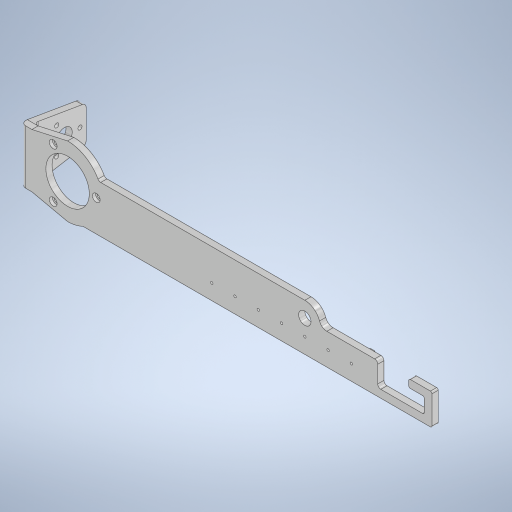
# Autodesk Inventor part: motor_holder_2
Saved by Autodesk Inventor 2024 (Build 280153000, 153)
## iProperties
Created: 2025-02-07
Part Number: motor_holder_2
Material: アルミニウム 6061
Document SubType Name: Modeling
Designer: 1412z
Density: 2.7 g/cm^3
Appearance: アルミニウム - つや出し
Author: 1412z
Autodesk Inventor part; units mm, degrees
ref_plane "YZ Plane" through (0, 0, 0) normal (1, 0, 0) x (0, 1, 0)
ref_plane "XZ Plane" through (0, 0, 0) normal (0, 1, 0) x (-1, 0, 0)
ref_plane "XY Plane" through (0, 0, 0) normal (0, 0, 1) x (1, 0, 0)
sketch "スケッチ1" plane through (0, 0, 0) normal (1, 0, 0) x (0, 1, 0)
  circle A0 centre (0, 0) radius 10
  circle A1 centre (0, -10) radius 1.35
  circle A2 centre (8.6603, 5) radius 1.35
  circle A3 centre (-8.6603, 5) radius 1.35
  circle A4 centre (0, 0) radius 5
  line L0 (0, 0) -> (0, 50)
  circle A5 centre (0, 50) radius 22.5
  circle A6 centre (0, 0) radius 14
  line L1 (-14, 0) -> (-22.5, 50)
  line L2 (14, 0) -> (22.5, 50)
  line L3 (0, -14) -> (-11.62, -14)
  line L4 (-11.62, -14) -> (-14, 0)
  line L5 (0, -14) -> (11.62, -14)
  line L6 (11.62, -14) -> (14, 0)
  line L7 (0, 20) -> (-17.4, 20)
  line L8 (0, 20) -> (17.4, 20)
  dimension "d0" = 20
  dimension "d1" = 2.7
  dimension "d4" = 360
  dimension "d6" = 10
  dimension "d7" = 50
  dimension "d8" = 45
  dimension "d9" = 28
  constraints: 18 end point, 7 point on line, 6 centre point, 6 coincident, 5 point on circle, 1 horizontal, 1 perpendicular, 1 tangent, 1 vertical, 1 vertical alignment, 10 other
  measures "d1" diameter of A1
  measures "d6" diameter of A4
  measures "d7" distance of L0.start L0.end
  measures "d8" diameter of A5
  measures "d9" diameter of A6
extrude "押し出し1" add sketch "スケッチ1" along normal blind 4 contours A0 A1 A3 A2 | A6 L1 L7 L0 | L0 L8 L2 A6 | A6 L6 L4 | L6 L5 A6 | A6 L3 L4
sketch "スケッチ2" plane through (0, -17.4, 20) normal (0, 0, 1) x (1, 0, 0)
  line L0 (0, 17.4) -> (30, 17.4)
  circle A0 centre (30, 17.4) radius 22.5
  circle A1 centre (30, 17.4) radius 18.5
  circle A2 centre (30, 17.4) radius 14
  circle A3 centre (48.5, 17.4) radius 1.35
  circle A4 centre (20.75, 33.4215) radius 1.35
  circle A5 centre (20.75, 1.3785) radius 1.35
  line L1 (0, 29.02) -> (0, 34.8) projected
  line L2 (0, 0) -> (0, 5.78) projected
  line L3 (0, 34.8) -> (0, 0)
  line L4 (4, 29.02) -> (4, 34.8) projected
  line L5 (4, 34.8) -> (7, 34.8)
  line L6 (7, 34.8) -> (30, 39.9)
  line L7 (4, 0) -> (4, 5.78) projected
  line L8 (4, 0) -> (7, 0)
  line L9 (7, 0) -> (30, -5.1)
  line L10 (4, 0) -> (0, 0)
  line L11 (0, 34.8) -> (4, 34.8) projected
  line L12 (0, 0) -> (0, 34.8)
  line L13 (0, 34.8) -> (4, 34.8)
  dimension "d14" = 37
  dimension "d12" = 30
  dimension "d13" = 45
  dimension "d15" = 28
  dimension "d16" = 2.7
  dimension "d19" = 360
  dimension "d21" = 3
  dimension "d22" = 3
  constraints: 18 end point, 5 centre point, 4 horizontal, 3 coincident, 2 point on circle, 1 collinear, 1 horizontal alignment, 1 perpendicular, 1 vertical, 9 other
  measures "d12" distance of L0.start L0.end
  measures "d13" diameter of A0
  measures "d15" diameter of A2
  measures "d16" diameter of A3
  measures "d21" distance of L4.end L5.end
  measures "d22" distance of L7.start L8.end
extrude "押し出し2" add sketch "スケッチ2" along normal blind 4 contours L3 L1 L11 L5 L6 A0 L0 | L0 A0 L9 L8 L10 L2 L3 | A0 L6 L9 | A3 A1 A5 A4
fillet "フィレット1" radius 3 2 edges at (4, 0, 20) (0, 0, 24)
fillet "フィレット2" radius 3 2 edges at (2, -11.62, -14) (2, 11.62, -14)
sketch "スケッチ7" plane through (0, -17.4, 24) normal (0, 0, 1) x (1, 0, 0)
  circle A0 centre (30, 17.4) radius 14 projected
  line L0 (30, 17.4) -> (182.95, 17.4)
  line L1 (30, 17.4) -> (182.95, 17.4) construction
  circle A1 centre (182.95, 17.4) radius 4
  circle A2 centre (182.95, 17.4) radius 10
  line L2 (182.95, 27.4) -> (50.1556, 27.4)
  arc A3 (30, -5.1) -> (30, 39.9) centre (30, 17.4) ccw projected
  line L3 (182.95, 27.4) -> (315.7444, 27.4) construction
  line L4 (182.95, 7.4) -> (50.1556, 7.4)
  point P0 (0, 17.4)
  dimension "d55" = 152.95
  dimension "d56" = 0
  dimension "d57" = 8
  dimension "d58" = 20
  dimension "d59" = 180
  constraints: 10 end point, 4 horizontal, 4 point on circle, 2 centre point, 2 coincident, 2 collinear, 1 tangent
  measures "d55" distance of L0.start L0.end
  measures "d56" distance between parallel lines of L0 L1
  measures "d57" diameter of A1
  measures "d58" diameter of A2
  measures "d59" angle of L2 L3
extrude "押し出し7" add sketch "スケッチ7" against normal blind 4 contours A3 L2 A2 L0 | L0 A2 L4 A3 | A2
fillet "フィレット3" radius 2 2 edges at (50.1556, 10, 22) (50.1556, -10, 22)
sketch "スケッチ8" plane through (0, -17.4, 24) normal (0, 0, 1) x (1, 0, 0)
  circle A0 centre (20.75, 33.4215) radius 1.35 projected
  circle A1 centre (20.75, 33.4215) radius 2.5
  circle A2 centre (48.5, 17.4) radius 1.35 projected
  circle A3 centre (48.5, 17.4) radius 2.5
  circle A4 centre (20.75, 1.3785) radius 1.35 projected
  circle A5 centre (20.75, 1.3785) radius 2.5
  point P0 (0, 17.4)
  dimension "d63" = 5
  dimension "d64" = 5
  dimension "d65" = 5
  constraints: 3 centre point, 3 coincident
  measures "d63" diameter of A1
  measures "d64" diameter of A3
  measures "d65" diameter of A5
extrude "押し出し8" cut sketch "スケッチ8" against normal blind 2 contours A0 | A1 | A3 | A4 | A5
sketch "スケッチ9" plane through (0, -17.4, 24) normal (0, 0, 1) x (1, 0, 0)
  circle A0 centre (182.95, 17.4) radius 4 projected
  line L0 (182.95, 17.4) -> (182.95, -2.8)
  line L1 (182.95, -2.8) -> (229.95, -2.8)
  line L2 (229.95, -2.8) -> (229.95, 17.2)
  arc A1 (182.95, 7.4) -> (182.95, 27.4) centre (182.95, 17.4) ccw projected
  line L3 (229.95, -2.8) -> (264.95, -2.8)
  line L4 (264.95, -2.8) -> (264.95, 17.2)
  line L5 (264.95, 17.2) -> (249.95, 17.2)
  line L6 (249.95, 17.2) -> (249.95, 12.2)
  line L7 (182.95, -2.8) -> (39.9101, -2.8)
  arc A2 (30, -5.1) -> (49.6163, 6.3796) centre (30, 17.4) ccw projected
  circle A3 centre (30, 17.4) radius 14 projected
  circle A4 centre (30, 17.4) radius 22.5
  arc A5 (49.6163, 28.4204) -> (51.36, 27.4) centre (51.36, 29.4) ccw projected
  circle A6 centre (51.36, 29.4) radius 2
  line L8 (51.36, 27.4) -> (182.95, 27.4) projected
  line L9 (51.36, 27.4) -> (182.95, 27.4)
  circle A7 centre (182.95, 17.4) radius 10
  line L10 (229.95, 17.2) -> (192.948, 17.2)
  line L11 (249.95, 12.2) -> (259.95, 12.2)
  line L12 (259.95, 12.2) -> (259.95, 2.2)
  line L13 (259.95, 2.2) -> (229.95, 2.2)
  point P0 (0, 17.4)
  point P1 (182.95, 7.4)
  point P2 (182.95, 27.4)
  point P3 (49.6163, 6.3796)
  dimension "d68" = 20.2
  dimension "d69" = 47
  dimension "d70" = 20
  dimension "d71" = 35
  dimension "d72" = 20
  dimension "d73" = 15
  dimension "d74" = 5
  dimension "d76" = 10
  dimension "d77" = 10
  constraints: 26 end point, 5 horizontal, 5 perpendicular, 3 coincident, 2 vertical, 1 centre point, 1 collinear, 1 point on circle, 1 point on line, 1 tangent, 7 other
  measures "d68" distance of L0.start L0.end
  measures "d69" distance of L0.end L1.end
  measures "d70" distance of L1.end L2.end
  measures "d71" distance of L1.end L3.end
  measures "d72" distance of L3.end L4.end
  measures "d73" distance of L4.end L5.end
  measures "d74" distance of L5.end L6.end
  measures "d76" distance of L6.end L11.end
  measures "d77" distance of L11.end L12.end
extrude "押し出し9" add sketch "スケッチ9" against normal blind 4 contours A1 L10 L2 L1 L0 | L0 L7 A2 A4 A5 L8 A7 | L2 L13 L12 L11 L6 L5 L4 L3
fillet "フィレット7" radius 5 1 edges at (192.948, -0.2, 22)
fillet "フィレット8" radius 2 2 edges at (39.9101, -20.2, 22) (229.95, -0.2, 22)
fillet "フィレット9" radius 2 1 edges at (229.95, -15.2, 22)
fillet "フィレット10" radius 1 6 edges at (249.95, -0.2, 22) (249.95, -5.2, 22) (259.95, -5.2, 22) (259.95, -15.2, 22) (264.95, -0.2, 22) (264.95, -20.2, 22)
sketch "スケッチ14" plane through (0, -17.4, 20) normal (0, 0, -1) x (-1, 0, 0)
  line L0 (-229.95, 15.2) -> (-229.95, 4.2) projected
  line L1 (-229.95, 7.1) -> (-229.95, 9.7)
  line L2 (-229.95, 9.7) -> (-117.95, 9.7)
  line L3 (-117.95, 9.7) -> (-117.95, 4.5)
  line L4 (-117.95, 4.5) -> (-229.95, 4.5)
  line L5 (-229.95, 4.5) -> (-229.95, 7.1)
  point P0 (0, 17.4)
  dimension "d116" = 2.6
  dimension "d117" = 112
  dimension "d118" = 5.2
  constraints: 10 end point, 2 perpendicular, 2 point on line, 1 collinear, 1 midpoint, 1 vertical
  measures "d116" distance of L1.start L1.end
  measures "d117" distance of L1.end L2.end
  measures "d118" distance of L2.end L3.end
extrude "押し出し14" cut sketch "スケッチ14" against normal blind 0.7
sketch "スケッチ18" plane through (0, -17.4, 20.7) normal (0, 0, -1) x (-1, 0, 0)
  circle A0 centre (-212.95, 7.1) radius 0.8
  circle A1 centre (-197.95, 7.1) radius 0.8
  circle A2 centre (-182.95, 7.1) radius 0.8
  circle A3 centre (-167.95, 7.1) radius 0.8
  circle A4 centre (-152.95, 7.1) radius 0.8
  circle A5 centre (-137.95, 7.1) radius 0.8
  circle A6 centre (-122.95, 7.1) radius 0.8
  point P0 (0, 17.4)
  dimension "d154" = 1.6
  dimension "d155" = 1.6
  dimension "d156" = 15
  dimension "d157" = 1.6
  dimension "d158" = 15
  dimension "d159" = 1.6
  dimension "d160" = 15
  dimension "d161" = 1.6
  dimension "d162" = 15
  dimension "d163" = 1.6
  dimension "d164" = 15
  dimension "d165" = 1.6
  dimension "d166" = 15
  constraints: 7 centre point
  measures "d154" diameter of A0
  measures "d155" diameter of A1
  measures "d156" distance between centres of A1 A0
  measures "d157" diameter of A2
  measures "d158" distance of A2.centre A1.centre
  measures "d159" diameter of A3
  measures "d160" distance of A3.centre A2.centre
  measures "d161" diameter of A4
  measures "d162" distance of A4.centre A3.centre
  measures "d163" diameter of A5
  measures "d164" distance of A5.centre A4.centre
  measures "d165" diameter of A6
  measures "d166" distance of A6.centre A5.centre
extrude "押し出し18" cut sketch "スケッチ18" against normal blind 10
sketch "スケッチ19" plane through (0, -17.4, 20.7) normal (0, 0, -1) x (-1, 0, 0)
  line L0 (-229.95, 4.5) -> (-229.95, 9.7) projected
  line L1 (-229.95, 4.5) -> (-225.15, 4.5)
  line L2 (-117.95, 4.5) -> (-229.95, 4.5) projected
  line L3 (-225.15, 4.5) -> (-225.15, 9.7)
  line L4 (-229.95, 9.7) -> (-117.95, 9.7) projected
  line L5 (-225.15, 9.7) -> (-229.95, 9.7)
  line L6 (-229.95, 9.7) -> (-229.95, 4.5)
  point P0 (0, 17.4)
  dimension "d169" = 4.8
  constraints: 8 end point, 2 perpendicular, 2 point on line, 1 horizontal
  measures "d169" distance of L0.start L1.end
extrude "押し出し19" add sketch "スケッチ19" along normal blind 0.7
sketch "スケッチ20" plane through (117.95, -12.9, 20) normal (1, 0, 0) x (0, 0, -1)
  line L0 (0, 5.2) -> (0, 0) projected
  line L1 (-0.7, 5.2) -> (-0.7, 0) projected
  line L2 (0, 0) -> (-0.7, 0)
  line L3 (-0.7, 0) -> (-0.7, 5.2)
  line L4 (0, 5.2) -> (-0.7, 5.2) projected
  line L5 (-0.7, 5.2) -> (0, 5.2)
  line L6 (0, 5.2) -> (0, 0)
  point P0 (20, 12.9)
  constraints: 8 end point, 2 collinear, 2 perpendicular
extrude "押し出し20" cut sketch "スケッチ20" against normal blind 0.2
sketch "スケッチ21" plane through (0, -17.4, 20) normal (0, 0, -1) x (-1, 0, 0)
  line L0 (-117.75, 4.5) -> (-225.15, 4.5) projected
  line L1 (-117.75, 4.5) -> (-117.75, -0.5)
  line L2 (-117.75, -0.5) -> (-114.75, -0.5)
  line L3 (-114.75, -0.5) -> (-114.75, 14.5)
  line L4 (-114.75, 14.5) -> (-117.75, 14.5)
  line L5 (-117.75, 14.5) -> (-117.75, 4.5)
  point P0 (0, 17.4)
  dimension "d174" = 5
  dimension "d175" = 3
  dimension "d176" = 15
  constraints: 10 end point, 3 perpendicular, 1 horizontal, 1 vertical
  measures "d174" distance of L0.start L1.end
  measures "d175" distance of L1.end L2.end
  measures "d176" distance of L2.end L3.end
extrude "押し出し21" add sketch "スケッチ21" along normal blind 3
fillet "フィレット13" radius 2 3 edges at (116.25, -17.9, 20) (114.75, -10.4, 20) (116.25, -2.9, 20)
sketch "スケッチ23" plane through (0, -17.4, 20.7) normal (0, 0, -1) x (-1, 0, 0)
  line L0 (-225.15, 9.7) -> (-225.15, 4.5) projected
  line L1 (-225.15, 9.7) -> (-218.15, 9.7)
  line L2 (-225.15, 9.7) -> (-117.75, 9.7) projected
  line L3 (-218.15, 9.7) -> (-218.15, 4.5)
  line L4 (-117.75, 4.5) -> (-225.15, 4.5) projected
  line L5 (-218.15, 4.5) -> (-225.15, 4.5)
  line L6 (-225.15, 4.5) -> (-225.15, 9.7)
  point P0 (0, 17.4)
  dimension "d185" = 7
  constraints: 8 end point, 2 perpendicular, 2 point on line, 1 collinear
  measures "d185" distance of L0.start L1.end
extrude "押し出し23" add sketch "スケッチ23" along normal blind 0.7
sketch "スケッチ26" plane through (0, -17.4, 20) normal (0, 0, -1) x (-1, 0, 0)
  line L0 (-218.15, 9.7) -> (-117.75, 9.7) projected
  line L1 (-218.15, 9.7) -> (-218.15, 14.7)
  line L2 (-218.15, 14.7) -> (-221.15, 14.7)
  line L3 (-221.15, 14.7) -> (-221.15, -0.3)
  line L4 (-221.15, -0.3) -> (-218.15, -0.3)
  line L5 (-218.15, -0.3) -> (-218.15, 9.7)
  point P0 (0, 17.4)
  dimension "d200" = 5
  dimension "d201" = 3
  dimension "d202" = 15
  constraints: 10 end point, 3 perpendicular, 1 collinear, 1 point on line, 1 vertical
  measures "d200" distance of L0.start L1.end
  measures "d201" distance of L1.end L2.end
  measures "d202" distance of L2.end L3.end
extrude "押し出し26" add sketch "スケッチ26" along normal blind 3
fillet "フィレット16" radius 2 3 edges at (219.65, -17.7, 20) (221.15, -10.2, 20) (219.65, -2.7, 20)
